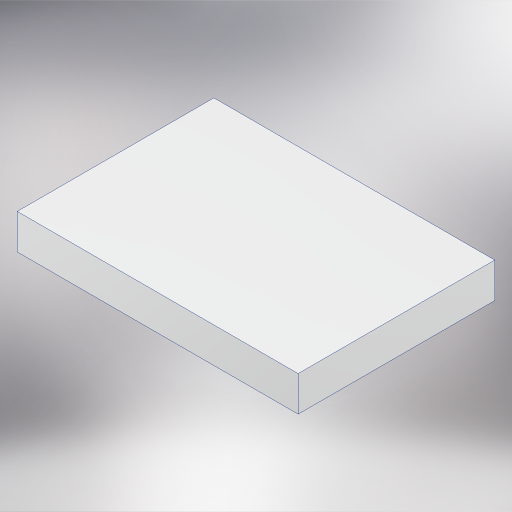
# Autodesk Inventor part: Heat Sink - V1
Saved by Autodesk Inventor 2024 (Build 280153000, 153)
## iProperties
Created: 2024-01-23
Part Number: Heat Sink - V1
Material: Aluminum 6061
Document SubType Name: Modeling
Designer: cfang
Density: 2.7 g/cm^3
Appearance: Aluminum - Flat
Author: cfang
Autodesk Inventor part; units mm, degrees
ref_plane "YZ Plane" through (0, 0, 0) normal (1, 0, 0) x (0, 1, 0)
ref_plane "XZ Plane" through (0, 0, 0) normal (0, 1, 0) x (-1, 0, 0)
ref_plane "XY Plane" through (0, 0, 0) normal (0, 0, 1) x (1, 0, 0)
sketch "Sketch1" plane through (0, 0, 0) normal (0, 1, 0) x (-1, 0, 0)
  line L0 (-20, 14) -> (20, 14)
  line L1 (20, 14) -> (20, -14)
  line L2 (20, -14) -> (-20, -14)
  line L3 (-20, -14) -> (-20, 14)
  line L4 (-20, 14) -> (20, -14) construction
  line L5 (20, 14) -> (-20, -14) construction
  point P0 (0, 0)
  dimension "d0" = 28
  dimension "d1" = 40
  constraints: 12 end point, 2 midpoint, 2 parallel, 1 horizontal, 1 perpendicular
  measures "d0" distance of L0.end L1.end
  measures "d1" distance of L0.start L0.end
extrude "Extrusion1" add sketch "Sketch1" along normal blind 5
body "Solid1"
